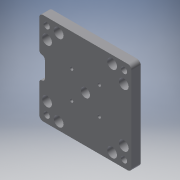
# Autodesk Inventor part: 20_IM_LED_holder
Saved by Autodesk Inventor 2019 (Build 230136000, 136)
## iProperties
Created: 2020-10-28
Part Number: 20_IM_LED_holder
Material: Generic
Document SubType Name: Modeling
Designer: wanghaoran
Density: 1 g/cm^3
Appearance: Default
Author: wanghaoran
Autodesk Inventor part; units mm, degrees
ref_plane "YZ Plane" through (0, 0, 0) normal (1, 0, 0) x (0, 1, 0)
ref_plane "XZ Plane" through (0, 0, 0) normal (0, 1, 0) x (-1, 0, 0)
ref_plane "XY Plane" through (0, 0, 0) normal (0, 0, 1) x (1, 0, 0)
sketch "Sketch1" plane through (0, 0, 0) normal (0, 0, 1) x (1, 0, 0)
  line L0 (-25, 25) -> (25, 25)
  line L1 (25, 25) -> (25, -25)
  line L2 (25, -25) -> (-25, -25)
  line L3 (-25, -25) -> (-25, 25)
  line L4 (-25, 25) -> (25, -25) construction
  line L5 (25, 25) -> (-25, -25) construction
  circle A0 centre (0, 0) radius 2.5
  circle A1 centre (-20.8, -14.5) radius 2.65
  circle A2 centre (-14.5, -20.8) radius 2.65
  circle A3 centre (-20.8, 14.5) radius 2.65
  circle A4 centre (20.8, -14.5) radius 2.65
  circle A5 centre (20.8, 14.5) radius 2.65
  circle A6 centre (-14.5, 20.8) radius 2.65
  circle A7 centre (14.5, -20.8) radius 2.65
  circle A8 centre (14.5, 20.8) radius 2.65
  dimension "d0" = 50
  dimension "d1" = 50
  dimension "d2" = 5
  dimension "d5" = 5.3
  dimension "d6" = 4.2
  dimension "d8" = 10.5
  dimension "d11" = 29
  dimension "d14" = 41.6
  constraints: 12 end point, 9 centre point, 4 symmetric about line, 2 horizontal, 2 midpoint, 2 parallel, 1 coincident, 1 perpendicular, 1 vertical, 10 other
  measures "d0" distance of L1.end L2.end
  measures "d1" distance of L0.end L1.end
  measures "d2" diameter of A0
  measures "d5" diameter of A1
  measures "d6" distance from line of A1.centre L3
  measures "d8" distance from line of L2 A1.centre
  measures "d11" distance of A1.centre A3.centre
  measures "d14" distance of A1.centre A4.centre
extrude "Extrusion1" add sketch "Sketch1" along normal blind 5
fillet "Fillet1" radius 2 4 edges at (-25, 25, 2.5) (25, 25, 2.5) (-25, -25, 2.5) (25, -25, 2.5)
sketch "Sketch2" plane through (0, 0, 5) normal (0, 0, 1) x (1, 0, 0)
  arc A0 (23, -25) -> (25, -23) centre (23, -23) ccw projected
  line L0 (25, -23) -> (25, 23) projected
  arc A1 (25, 23) -> (23, 25) centre (23, 23) ccw projected
  line L1 (23, 25) -> (-23, 25) projected
  arc A2 (-23, 25) -> (-25, 23) centre (-23, 23) ccw projected
  line L2 (-25, 23) -> (-25, -23) projected
  arc A3 (-25, -23) -> (-23, -25) centre (-23, -23) ccw projected
  line L3 (-23, -25) -> (23, -25) projected
  circle A4 centre (14.5, 20.8) radius 2.65 projected
  circle A5 centre (-14.5, 20.8) radius 2.65 projected
  circle A6 centre (14.5, -20.8) radius 2.65 projected
  circle A7 centre (20.8, 14.5) radius 2.65 projected
  circle A8 centre (20.8, -14.5) radius 2.65 projected
  circle A9 centre (-20.8, 14.5) radius 2.65 projected
  circle A10 centre (-14.5, -20.8) radius 2.65 projected
  circle A11 centre (-20.8, -14.5) radius 2.65 projected
  circle A12 centre (0, 0) radius 2.5 projected
  line L4 (21, -21) -> (-21, -21)
  line L5 (-21, -21) -> (-21, 21)
  line L6 (-21, 21) -> (21, 21)
  line L7 (21, 21) -> (21, -21)
  line L8 (21, -21) -> (-21, 21) construction
  line L9 (-21, -21) -> (21, 21) construction
  circle A13 centre (-28.6, 21.06) radius 1.55 projected
  dimension "d18" = 42
  dimension "d19" = 42
  constraints: 12 end point, 2 midpoint, 2 parallel, 1 horizontal, 1 perpendicular
  measures "d18" distance of L5.end L6.end
  measures "d19" distance of L4.end L5.end
hole "Hole1" at (-21, 21, 5) at (21, 21, 5) at (21, -21, 5) at (-21, -21, 5) direction (0, 0, -1) diameter 3.3 end through all both
sketch "Sketch3" plane through (0, 0, 0) normal (0, 0, -1) x (-1, 0, 0)
  circle A0 centre (-21, -21) radius 1.65 construction
  circle A1 centre (21, 21) radius 1.65 construction
  circle A2 centre (-21, 21) radius 1.65 construction
  circle A3 centre (21, -21) radius 1.65 construction
  circle A4 centre (-14.5, 20.8) radius 2.65 construction
  circle A5 centre (14.5, 20.8) radius 2.65 construction
  circle A6 centre (-14.5, -20.8) radius 2.65 construction
  circle A7 centre (-20.8, 14.5) radius 2.65 construction
  circle A8 centre (-20.8, -14.5) radius 2.65 construction
  circle A9 centre (20.8, 14.5) radius 2.65 construction
  circle A10 centre (14.5, -20.8) radius 2.65 construction
  circle A11 centre (20.8, -14.5) radius 2.65 construction
  circle A12 centre (0, 0) radius 2.5 construction
  arc A13 (-25, -23) -> (-23, -25) centre (-23, -23) ccw construction
  line L0 (-23, -25) -> (23, -25) construction
  arc A14 (23, -25) -> (25, -23) centre (23, -23) ccw construction
  line L1 (25, -23) -> (25, 23) construction
  arc A15 (25, 23) -> (23, 25) centre (23, 23) ccw construction
  line L2 (23, 25) -> (-23, 25) construction
  arc A16 (-23, 25) -> (-25, 23) centre (-23, 23) ccw construction
  line L3 (-25, 23) -> (-25, -23) construction
  circle A17 centre (-7.5, 7.5) radius 0.9 construction
  circle A18 centre (7.5, 7.5) radius 0.9 construction
  circle A19 centre (7.5, -7.5) radius 0.9 construction
  circle A20 centre (-7.5, -7.5) radius 0.9 construction
  constraints: 4 centre point, 8 other
hole "Hole2" at (7.5, 7.5, 0) at (-7.5, 7.5, 0) at (-7.5, -7.5, 0) at (7.5, -7.5, 0) direction (0, 0, 1) diameter 1.8 end through all
sketch "Sketch4" plane through (0, 0, 0) normal (0, 0, -1) x (-1, 0, 0)
  line L0 (15, 15) -> (15, -15) construction
  line L1 (-15, 15) -> (15, 15) construction
  line L2 (15, -15) -> (-15, -15) construction
  line L3 (-15, -15) -> (-15, 15) construction
  circle A0 centre (7.5, -7.5) radius 0.9 construction
  circle A1 centre (-7.5, 7.5) radius 0.9 construction
  circle A2 centre (7.5, 7.5) radius 0.9 construction
  circle A3 centre (-7.5, -7.5) radius 0.9 construction
  circle A4 centre (-21, -21) radius 1.65 construction
  circle A5 centre (21, 21) radius 1.65 construction
  circle A6 centre (-21, 21) radius 1.65 construction
  circle A7 centre (21, -21) radius 1.65 construction
  circle A8 centre (-14.5, 20.8) radius 2.65 construction
  circle A9 centre (14.5, 20.8) radius 2.65 construction
  circle A10 centre (-14.5, -20.8) radius 2.65 construction
  circle A11 centre (-20.8, 14.5) radius 2.65 construction
  circle A12 centre (-20.8, -14.5) radius 2.65 construction
  circle A13 centre (20.8, 14.5) radius 2.65 construction
  circle A14 centre (14.5, -20.8) radius 2.65 construction
  circle A15 centre (20.8, -14.5) radius 2.65 construction
  circle A16 centre (0, 0) radius 2.5 construction
  arc A17 (-25, -23) -> (-23, -25) centre (-23, -23) ccw construction
  line L4 (-23, -25) -> (23, -25) construction
  arc A18 (23, -25) -> (25, -23) centre (23, -23) ccw construction
  line L5 (25, -23) -> (25, 23) construction
  arc A19 (25, 23) -> (23, 25) centre (23, 23) ccw construction
  line L6 (23, 25) -> (-23, 25) construction
  arc A20 (-23, 25) -> (-25, 23) centre (-23, 23) ccw construction
  line L7 (-25, 23) -> (-25, -23) construction
  line L8 (-25, -23) -> (-25, 23) construction
  line L9 (-25, 0) -> (25, 0) construction
  line L10 (25, 23) -> (25, -23) construction
  line L11 (10, 6) -> (15, 6) construction
  line L12 (15, 6) -> (15, -6) construction
  line L13 (15, -6) -> (10, -6) construction
  line L14 (10, -6) -> (10, 6) construction
  line L15 (10, 6) -> (25, 6)
  line L16 (25, 6) -> (25, -6)
  line L17 (25, -6) -> (10, -6)
  line L18 (10, -6) -> (10, 6)
  dimension "d34" = 5
  dimension "d35" = 12
  constraints: 26 end point, 4 horizontal, 4 parallel, 2 midpoint, 2 perpendicular, 2 point on line, 2 vertical, 1 collinear, 5 other
  measures "d34" distance of L11.start L11.end
  measures "d35" distance of L13.end L11.start
extrude "Extrusion2" cut sketch "Sketch4" against normal blind 3
sketch "Sketch5" plane through (0, 0, 3) normal (0, 0, -1) x (-1, 0, 0)
  line L0 (10, 6) -> (25, 6) projected
  line L1 (10, -6) -> (10, 6) projected
  line L2 (25, -6) -> (10, -6) projected
  line L3 (25, 6) -> (25, -6) projected
  line L4 (25, 6) -> (25, -6) projected
  line L5 (25, -6) -> (10, -6) projected
  line L6 (25, 6) -> (22, 6)
  line L7 (22, 6) -> (22, -6)
  line L8 (22, -6) -> (25, -6)
  line L9 (25, -6) -> (25, 6)
  point P0 (0, 0)
  dimension "d38" = 3
  constraints: 8 end point, 2 parallel, 1 horizontal, 1 perpendicular, 1 point on line
  measures "d38" distance between parallel lines of L3 L7
extrude "Extrusion3" cut sketch "Sketch5" against normal up to surface (2 mm away) contours L0 L3 L2 L7
fillet "Fillet2" radius 1.5 4 edges at (-25, 6, 2.5) (-25, -6, 2.5) (-22, 6, 4) (-22, -6, 4)
body "Solid1"
